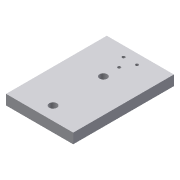
# Autodesk Inventor part: plinth
Saved by Autodesk Inventor 2016 (Build 200138000, 138)
## iProperties
Created: 2014-03-11
Part Number: plinth
Material: Concrete
Document SubType Name: Modeling
Designer: Dave
Density: 2.40731 g/cm^3
Appearance: Exposed Aggregate - Coarse
Mass: 77996.9 g
Surface Area: 17640 cm^2
Volume: 32400 cm^3
Author: Dave
Autodesk Inventor part; units mm, degrees
ref_plane "YZ Plane" through (0, 0, 0) normal (1, 0, 0) x (0, 1, 0)
ref_plane "XZ Plane" through (0, 0, 0) normal (0, 1, 0) x (-1, 0, 0)
ref_plane "XY Plane" through (0, 0, 0) normal (0, 0, 1) x (1, 0, 0)
sketch "Sketch1" plane through (0, 0, 0) normal (0, 1, 0) x (-1, 0, 0)
  line L0 (0, 0) -> (1000, 0)
  line L1 (1000, 0) -> (1000, 1500)
  line L2 (1000, 1500) -> (0, 1500)
  line L3 (0, 1500) -> (0, 0)
  dimension "d0" = 1000
  dimension "d1" = 1500
  constraints: 8 end point, 2 parallel, 1 horizontal, 1 perpendicular
  measures "d0" distance of L2.end L1.end
  measures "d1" distance of L2.end L0.start
extrude "base" add sketch "Sketch1" along normal blind 150
sketch "Sketch2" plane through (0, 150, 0) normal (0, 1, 0) x (1, 0, 0)
  circle A0 centre (-500, -550) radius 57.5
  line L0 (0, 0) -> (-1000, 0) projected
  line L1 (-1000, -1500) -> (0, -1500) projected
  line L2 (-500, 0) -> (-500, -1500) construction
  dimension "d4" = 115
  dimension "d38" = 550
  constraints: 2 end point, 2 midpoint, 1 centre point, 1 point on line
  measures "d4" diameter of A0
  measures "d38" distance from line of A0.centre L0
extrude "air" cut sketch "Sketch2" against normal through all
sketch "Sketch3" plane through (0, 150, 0) normal (0, 1, 0) x (1, 0, 0)
  circle A0 centre (-500, -550) radius 57.5 projected
  circle A1 centre (-400, -150) radius 22.5
  circle A2 centre (-600, -150) radius 22.5
  dimension "d7" = 45
  dimension "d39" = 400
  dimension "d40" = 100
  dimension "d41" = 45
  dimension "d42" = 100
  dimension "d43" = 400
  constraints: 2 centre point
  measures "d7" diameter of A1
  measures "d39" vertical distance of A0.centre A1.centre
  measures "d40" horizontal distance of A0.centre A1.centre
  measures "d41" diameter of A2
  measures "d42" horizontal distance of A2.centre A0.centre
  measures "d43" vertical distance of A2.centre A0.centre
extrude "power" cut sketch "Sketch3" against normal blind 254 contours A1 | A2
sketch "Sketch4" plane through (0, 150, 0) normal (0, 1, 0) x (1, 0, 0)
  circle A0 centre (-600, -150) radius 22.5 projected
  circle A1 centre (-500, -315) radius 22.5
  line L0 (0, 0) -> (-1000, 0) projected
  dimension "d52" = 45
  dimension "d53" = 315
  constraints: 1 centre point
  measures "d52" diameter of A1
  measures "d53" distance from line of A1.centre L0
hole "fibre" at (-500, 150, 315) direction (0, -1, 0) diameter 45 end through all
sketch "Sketch6" plane through (0, 150, 0) normal (0, 1, 0) x (1, 0, 0)
  circle A0 centre (-500, -550) radius 57.5 projected
  circle A1 centre (-500, -1300) radius 76.2
  dimension "d29" = 152.4
  dimension "d30" = 750
  constraints: 1 centre point
  measures "d29" diameter of A1
  measures "d30" distance of A1.centre A0.centre
hole "air2" at (-500, 150, 1300) direction (0, -1, 0) diameter 115 end through all
body "Solid1"
